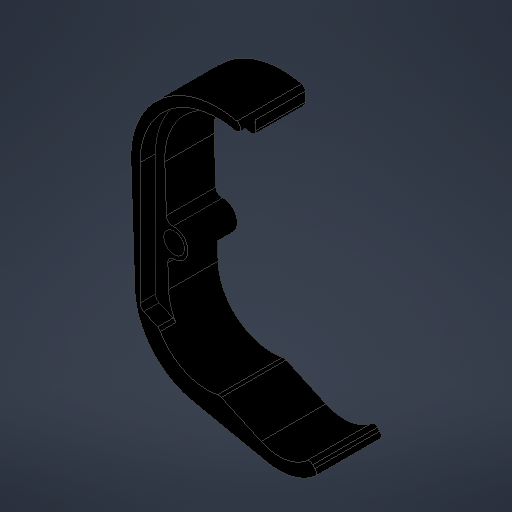
# Autodesk Inventor part: Dribbler Cover
Saved by Autodesk Inventor 2026.1 (Build 301233020, 233B)
## iProperties
Created: 2026-02-15
Part Number: Dribbler Cover
Material: Generic
Document SubType Name: Modeling
Designer: Bahaa
Density: 1 g/cm^3
Appearance: Default
Author: Bahaa
Autodesk Inventor part; units mm, degrees
ref_plane "YZ Plane" through (0, 0, 0) normal (1, 0, 0) x (0, 1, 0)
ref_plane "XZ Plane" through (0, 0, 0) normal (0, 1, 0) x (-1, 0, 0)
ref_plane "XY Plane" through (0, 0, 0) normal (0, 0, 1) x (1, 0, 0)
derived "Dribbler Bracket.ipt"
sketch "Sketch1" plane through (0, 0, 0) normal (0, 1, 0) x (-1, 0, 0)
  circle A0 centre (0, 0) radius 1.75
  circle A1 centre (10, 11.472) radius 12
  line L0 (0, 0) -> (10, 11.472) construction
  line L1 (0, 0) -> (4, 0) construction
  circle A2 centre (0, 0) radius 4
  circle A3 centre (0, -11.4408) radius 6.5
  line L2 (10, 11.472) -> (0, -11.4408) construction
  line L3 (0, 0) -> (0, -11.4408) construction
  line L4 (0, 0) -> (0, -4) construction
  line L5 (22, 11.472) -> (22, -8.528)
  line L6 (22, -8.528) -> (2.7031, -17.3521)
  line L7 (-2, 11.472) -> (-2, 6.472)
  line L8 (-2, 6.472) -> (-6.2853, -9.784)
  circle A4 centre (10, 11.472) radius 9.55
  line L9 (10, 11.472) -> (17.5, 11.472) construction
  circle A5 centre (17.5, 11.472) radius 1.1
  circle A6 centre (6.25, 17.9672) radius 1.1
  circle A7 centre (6.25, 4.9768) radius 1.1
  circle A8 centre (10, 11.472) radius 6.1
  circle A9 centre (0, -11.4408) radius 4.025
  circle A10 centre (10, 11.472) radius 10
  circle A11 centre (0, -11.4408) radius 5
  circle A12 centre (11.6246, -6.2035) radius 7.75
  circle A13 centre (11.6246, -6.2035) radius 4.025
  circle A14 centre (19, -5.528) radius 1.6
  circle A15 centre (19.5, 0.472) radius 1.35
  circle A16 centre (19.5, 0.472) radius 2.25
  circle A17 centre (10, 11.472) radius 11
  circle A18 centre (11.6246, -6.2035) radius 8.75
  line L10 (20.9931, 11.0822) -> (20.3691, -6.5135)
  circle A19 centre (0, -11.4408) radius 6
  line L11 (13.4136, -14.7686) -> (1.2267, -17.3141)
  line L12 (14.027, -17.7052) -> (1.8401, -20.2507)
  circle A20 centre (11.6246, -6.2035) radius 11.75
  line L13 (23.9912, 10.9759) -> (23.3673, -6.6199)
  circle A21 centre (10, 11.472) radius 14
  circle A22 centre (0, -11.4408) radius 9
  line L14 (6.25, 21.8131) -> (6.25, 24.9605)
  line L15 (0, -11.4408) -> (-14.1421, -25.583)
  line L16 (0, -11.4408) -> (20, -11.4408) construction
  line L17 (2.9111, -17.8068) -> (22.5, -8.8491)
  line L18 (22.5, -8.8491) -> (22.5, 11.472)
  circle A23 centre (0, -11.4408) radius 7
  circle A24 centre (10, 11.472) radius 12.5
  circle A25 centre (0, -11.4408) radius 5.5
  circle A26 centre (10, 11.472) radius 10.5
  point P0 (-3.9182, -0.8047)
  point P1 (-3.0124, 2.6317)
  point P2 (3.3685, 2.1571)
  point P3 (2.9717, 1.7457)
  point P4 (3.8203, 1.1856)
  point P5 (4.0975, -16.7145)
  point P6 (-4.5962, -16.037)
  point P7 (-6.364, -17.8048)
  point P8 (1.8401, -20.2507)
  point P9 (23.3673, -6.6199)
  point P10 (23.9912, 10.9759)
  point P11 (20.6847, 2.3849)
  point P12 (20.5462, -1.5199)
  point P13 (20.4296, -4.8094)
  point P14 (20.3751, -6.346)
  point P15 (-4.2426, -15.6835)
  point P16 (6.3108, -16.2522)
  point P17 (6.25, 23.3963)
  point P18 (-4.9497, -16.3906)
  point P19 (19.3658, -10.2824)
  point P20 (9.6463, -14.7269)
  dimension "d17" = 4.5
  dimension "d18" = 1
  dimension "d19" = 1
  dimension "d20" = 1
  dimension "d22" = 3
  dimension "d23" = 3
  dimension "d24" = 3
  dimension "d25" = 3
  dimension "d26" = 3
  dimension "d27" = 20
  dimension "d28" = 135
  dimension "d29" = 0.5
  dimension "d30" = 0.5
  dimension "d31" = 0.5
  measures "d17" diameter of A16
  measures "d18" radial gap between concentric circles of A10 A17
  measures "d19" radial gap between concentric circles of A12 A18
  measures "d22" distance between parallel lines of L11 L12
  measures "d23" radial gap between concentric circles of A18 A20
  measures "d24" distance between parallel lines of L10 L13
  measures "d27" distance of L15.start L15.end
  measures "d28" angle of L15 L16
  measures "d29" distance between parallel lines of L6 L17
  measures "d30" radial gap between concentric circles of A3 A23
  measures "d31" radial gap between concentric circles of A1 A24
extrude "Extrusion1" add sketch "Sketch1" along normal blind 8 contours A21 L18 A24 L14 | L15 A23 L17 A20 A22 | A24 L5 A1 L14 | A22 A20 L12 | A1 L10 A17 L14 | L18 A21 L5 A24 | L13 A20 L18 A21 | A20 A22 L11 A18 L17 L18 | A20 L17 L11 A22 | L5 A24 L10 A1 | L18 A20 L5 A21 | L5 A21 L10 A24 | A22 L17 A18 L11 | L11 L17 A22 | L5 A20 A16 L10 A21 | L18 L17 A18 L6 L5 A20 | A21 A18 A16 | A16 A18 A21 | A16 A24 A20 A21 A15 A18 | A16 A24 | L5 L6 A18 A14 L10 A16 A20 | A18 A21 A15 L10 A16 | A20 L10 A16 | A16 L10 A15 A20 | L10 A20 A21 A16 | A21 A20 A16 | A14 L10 | A21 A15 L10 | A15 A21 | L10 A15 A21 A20 | L10 A15
hole "Hole1" at (-19.5, 0, 0.472) direction (0, 1, 0) diameter 3.3 depth 4
extrude "Extrusion2" add sketch "Sketch1" against normal blind 2.5 contours A21 L18 A24 L14 | L15 A23 L17 A20 A22 | A22 A20 L12 | L13 A20 L18 A21 | A20 A22 L11 A18 L17 L18 | A20 L17 L11 A22 | A22 L17 A18 L11 | L11 L17 A22
fillet "Fillet1" radius 1 5 edges at (-20.6847, 4, 2.3849) (-20.5462, 4, -1.5199) (-9.6463, 2.75, -14.7269) (-22.5, -1.25, -8.8491) (-19.3658, -1.25, -10.2824)
fillet "Fillet2" radius 0.75 5 edges at (-6.25, 2.75, 24.9605) (-6.25, 4, 21.8131) (4.9497, 2.75, -16.3906) (6.364, 2.75, -17.8048) (-6.25, -1.25, 23.3963)
body "Solid1"
